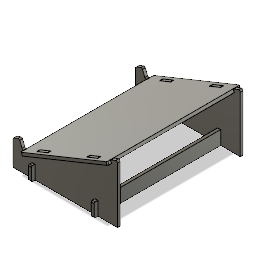
Laptop Stand v2 (Autodesk Fusion 360 design; units mm, degrees)
Autodesk Fusion 360 part; units mm, degrees
sketch "Sketch1" plane through (0, 0, 0) normal (0, 0, 1) x (1, 0, 0) in component "Leg1"
  line L0 (0, 55) -> (0, 0)
  line L1 (0, 0) -> (225, 0)
  line L2 (225, 0) -> (225, 125)
  line L3 (225, 125) -> (21.2612, 42.6842)
  line L4 (21.2612, 42.6842) -> (14, 60.6564)
  line L5 (14, 60.6564) -> (0, 55)
  dimension "d1" = 225
  dimension "d2" = 55
  dimension "d3" = 14
  dimension "d4" = 22
  dimension "d5" = 125
  measures "d1" distance of L0.end
  measures "d3" distance of L0.end
  measures "d4" angle of L1 L3
  measures "d5" distance of L0.end
extrude "Extrude1" add sketch "Sketch1" along normal blind 6.35 makes body 1 in component "Leg1"
fillet "Fillet1" radius 3 4 edges at (0, 0, 3.175) (0, 55, 3.175) (14, 60.6564, 3.175) (21.2612, 42.6842, 3.175) on bodies 1 in component "Leg1"
sketch "Sketch2" plane through (51.4611, -0.7369, 6.35) normal (0, 0, 1) x (1, 0, 0) in component "Leg1"
  arc A0 (-36.3373, 58.6117) -> (-40.2427, 60.2695) centre (-39.1189, 57.4879) ccw
  line L0 (-40.2427, 60.2695) -> (-49.585, 56.4949)
  arc A1 (-49.585, 56.4949) -> (-51.4611, 53.7134) centre (-48.4611, 53.7134) ccw
  line L1 (-51.4611, 53.7134) -> (-51.4611, 3.7369)
  arc A2 (-51.4611, 3.7369) -> (-48.4611, 0.7369) centre (-48.4611, 3.7369) ccw
  line L2 (-48.4611, 0.7369) -> (173.5389, 0.7369)
  line L3 (173.5389, 0.7369) -> (173.5389, 125.7369)
  line L4 (173.5389, 125.7369) -> (-27.4184, 44.5449)
  arc A3 (-31.3237, 46.2027) -> (-27.4184, 44.5449) centre (-28.5422, 47.3265) ccw
  line L5 (-31.3237, 46.2027) -> (-36.3373, 58.6117)
move_body "Move1" bodies 1 to x (1, 0, 0) y (0, 1, 0) z (0, 0, 1) at (0, 0, 270) in component "Leg1"
extrude "Extrude2" add sketch "Sketch2" along normal blind 6.35 separate body makes body 2 in component "Leg1"
fillet "Fillet2" radius 3 2 edges at (225, 125, 273.175) (225, 125, 9.525) on bodies 1 2 in component "Leg1"
sketch "Sketch6" plane through (-11.8419, 29.3097, 0) normal (-0.374607, 0.927184, 0) x (0, 0, 1) in component "Leg1"
  line L0 (12.7, 250.9945) -> (6.35, 250.9945)
  line L1 (6.35, 250.9945) -> (6.35, 38.7028)
  line L2 (6.35, 38.7028) -> (12.7, 38.7028)
  line L3 (12.7, 38.7028) -> (12.7, 250.9945)
sketch "Sketch4" plane through (-11.8419, 29.3097, 0) normal (-0.374607, 0.927184, 0) x (0, 0, 1) in component "Top1"
  line L0 (276.35, 250.9945) -> (270, 250.9945)
  line L1 (270, 250.9945) -> (270, 38.7028)
  line L2 (270, 38.7028) -> (276.35, 38.7028)
  line L3 (276.35, 38.7028) -> (276.35, 250.9945)
  line L4 (-1.65, 238.9945) -> (284.35, 238.9945)
  line L5 (284.35, 238.9945) -> (284.35, 38.7028)
  line L6 (284.35, 38.7028) -> (-1.65, 38.7028)
  line L7 (-1.65, 38.7028) -> (-1.65, 238.9945)
  line L8 (6.35, 250.9945) -> (6.35, 38.7028)
  line L9 (270, 208.9945) -> (276.35, 208.9945)
  line L10 (276.35, 208.9945) -> (276.35, 183.9945)
  line L11 (276.35, 183.9945) -> (270, 183.9945)
  line L12 (270, 183.9945) -> (270, 208.9945)
  line L13 (141.35, 238.9945) -> (141.35, 38.7028)
  line L14 (-1.65, 138.8487) -> (284.35, 138.8487)
  line L15 (141.35, 38.7028) -> (141.35, 238.9945)
  line L16 (270, 93.7028) -> (270, 68.7028)
  line L17 (270, 68.7028) -> (276.35, 68.7028)
  line L18 (276.35, 68.7028) -> (276.35, 93.7028)
  line L19 (276.35, 93.7028) -> (270, 93.7028)
  line L20 (6.35, 208.9945) -> (6.35, 183.9945)
  line L21 (12.7, 208.9945) -> (6.35, 208.9945)
  line L22 (12.7, 183.9945) -> (12.7, 208.9945)
  line L23 (6.35, 183.9945) -> (12.7, 183.9945)
  line L24 (6.35, 93.7028) -> (12.7, 93.7028)
  line L25 (6.35, 68.7028) -> (6.35, 93.7028)
  line L26 (12.7, 93.7028) -> (12.7, 68.7028)
  line L27 (12.7, 68.7028) -> (6.35, 68.7028)
  dimension "d14" = 12
  dimension "d15" = 8
  dimension "d16" = 8
  dimension "d17" = 25
  dimension "d18" = 30
  measures "d14" distance of L0 L4
  measures "d15" distance of L3 L5
  measures "d16" distance of L7 L8
  measures "d17" distance of L9 L11
  measures "d18" distance of L4 L9
extrude "Extrude3" add sketch "Sketch4" against normal blind 6.35 separate body contours L3 L4 L5 L10 L14 | L1 L3 L4 L9 | L1 L4 L12 L13 L14 L15 | L4 L8 L13 L14 L15 L21 L22 L23 | L1 L3 L11 L14 | L3 L5 L6 L14 L18 | L4 L7 L8 L14 L20 | L1 L6 L13 L14 L15 L16 | L6 L8 L13 L14 L15 L24 L26 L27 | L1 L3 L14 L19 | L6 L7 L8 L14 L25 | L1 L2 L3 L6 L17 makes body 3 in component "Top1"
combine "Combine2" operation cut target body 1 tool bodies 3 keep tools in component "Leg1"
combine "Combine3" operation cut target body 2 tool bodies 3 keep tools in component "Leg1"
fillet "Fillet1'" radius 2 4 edges at (25.2322, 40.8642, -1.65) (25.2322, 40.8642, 284.35) (210.9393, 115.8948, -1.65) (210.9393, 115.8948, 284.35) on bodies 3 in component "Top1"
ref_plane "WorkPlane1" through (180, 60.2762, 273.175) normal (1, 0, 0) x (0, 1, 0) in component "Support 1"
sketch "Sketch1 (2)" plane through (180, 60.2762, 273.175) normal (1, 0, 0) x (0, 0, -1) in component "Support 1"
ref_plane "WorkPlane2" through (180, 60.2762, 273.175) normal (1, 0, 0) x (0, 1, 0) in component "Support 1"
sketch "Sketch4 (2)" plane through (180, 60.2762, 273.175) normal (1, 0, 0) x (0, 0, -1) in component "Support 1"
  line L0 (260.475, 46.5427) -> (260.475, -60.2762)
  line L1 (260.475, -60.2762) -> (266.825, -60.2762)
  line L2 (266.825, -60.2762) -> (266.825, 46.5427)
  line L3 (266.825, 46.5427) -> (260.475, 46.5427)
  line L4 (3.175, 46.5427) -> (-3.175, 46.5427)
  line L5 (-3.175, 46.5427) -> (-3.175, -60.2762)
  line L6 (-3.175, -60.2762) -> (3.175, -60.2762)
  line L7 (3.175, -60.2762) -> (3.175, 46.5427)
  line L8 (-11.175, -60.2762) -> (274.825, -60.2762)
  line L9 (274.825, -60.2762) -> (274.825, -30.2762)
  line L10 (274.825, -30.2762) -> (-11.175, -30.2762)
  line L11 (-11.175, -30.2762) -> (-11.175, -60.2762)
  line L12 (274.825, -21.6065) -> (274.825, 51.9256)
  line L13 (-11.175, 51.9256) -> (-11.175, -21.6065)
  line L14 (-11.175, -45.2762) -> (274.825, -45.2762)
  dimension "d24" = 286
  dimension "d25" = 30
  measures "d24" distance of origin
extrude "Extrude1'" add sketch "Sketch4 (2)" along normal mid plane 6.35 separate body contours L0 L7 L10 L14 | L0 L1 L2 L8 L14 | L0 L7 L8 L14 | L2 L9 L10 L14 | L5 L6 L7 L8 L14 | L2 L8 L9 L14 | L5 L10 L11 L14 | L5 L8 L11 L14 makes body 4 in component "Support 1"
ref_plane "WorkPlane3" through (112.5, 60.2762, 273.175) normal (1, 0, 0) x (0, 1, 0) in component "Support 1"
ref_plane "WorkPlane4" through (112.5, 60.2762, 273.175) normal (1, 0, 0) x (0, 1, 0) in component "Support 1"
fillet "Fillet1''" radius 2 4 edges at (180, 0, -1.65) (180, 0, 284.35) (180, 30, -1.65) (180, 30, 284.35) on bodies 4 in component "Support 1"
fillet "Fillet2'" radius 0.5 4 edges at (180, 30, 276.35) (180, 30, 12.7) (180, 30, 270) (180, 30, 6.35) on bodies 4 in component "Support 1"
mirror "Mirror1" about plane through (112.5, 60.2762, 273.175) normal (1, 0, 0) of bodies 4 makes body 5 in component "Support 1"
combine "Combine4" operation cut target body 1 tool bodies 5 4 keep tools in component "Leg1"
combine "Combine5" operation cut target body 2 tool bodies 4 5 keep tools in component "Leg1"
fillet "Fillet3" radius 0.5 4 edges at (183.175, 0, 9.525) (176.825, 0, 9.525) (41.825, 0, 9.525) (48.175, 0, 9.525) on bodies 2 in component "Leg1"
fillet "Fillet4" radius 0.5 4 edges at (41.825, 0, 273.175) (48.175, 0, 273.175) (176.825, 0, 273.175) (183.175, 0, 273.175) on bodies 1 in component "Leg1"
fillet "Fillet5" radius 0.5 6 edges at (24.0428, 43.808, 9.525) (51.8583, 55.0462, 9.525) (75.0379, 64.4114, 9.525) (158.7549, 98.2352, 9.525) (181.9345, 107.6004, 9.525) (209.75, 118.8386, 9.525) on bodies 2 in component "Leg1"
fillet "Fillet6" radius 0.5 6 edges at (24.0428, 43.808, 273.175) (51.8583, 55.0462, 273.175) (75.0379, 64.4114, 273.175) (158.7549, 98.2352, 273.175) (181.9345, 107.6004, 273.175) (209.75, 118.8386, 273.175) on bodies 1 in component "Leg1"
component "Leg1" placed x (1, 0, 0) y (0, 1, 0) z (0, 0, 1) at (0, 0, 0)
component "Top1" placed x (1, 0, 0) y (0, 1, 0) z (0, 0, 1) at (0, 0, 0)
component "Support 1" placed x (1, 0, 0) y (0, 1, 0) z (0, 0, 1) at (0, 0, 0)
equation "t = 0.25 in"
equation "legWidth = 270 mm"
equation "d8 = t"
equation "d11 = t"
equation "d19 = -t"
equation "d26 = t / 2"
